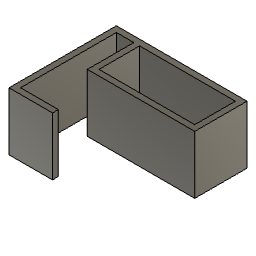
hook for a tee part 2 (Autodesk Fusion 360 design; units mm, degrees)
Autodesk Fusion 360 part; units mm, degrees
sketch "Sketch1" plane through (0, 0, 0) normal (0, 0, 1) x (1, 0, 0)
  line L0 (0, 0) -> (33, 0)
  line L1 (33, 0) -> (33, 14)
  line L2 (33, 14) -> (0, 14)
  line L3 (0, 14) -> (0, 0)
  line L4 (-2, 16) -> (35, 16)
  line L5 (35, 16) -> (35, -2)
  line L6 (35, -2) -> (-2, -2)
  line L7 (-2, -2) -> (-2, 16)
  line L8 (-2, 14) -> (-10, 14)
  line L9 (-10, 14) -> (-10, 16)
  line L10 (-10, 16) -> (-2, 16)
  line L11 (-2, 16) -> (-2, 14)
  line L12 (-10, 14) -> (-8, 14)
  line L13 (-8, 14) -> (-8, -19)
  line L14 (-8, -19) -> (-10, -19)
  line L15 (-10, -19) -> (-10, 14)
  line L16 (-10, -19) -> (5, -19)
  line L17 (5, -19) -> (5, -21)
  line L18 (5, -21) -> (-10, -21)
  line L19 (-10, -21) -> (-10, -19)
  dimension "d1" = 33
  dimension "d2" = 14
  dimension "d3" = 33
  dimension "d4" = 15
  dimension "d5" = 2
  constraint horizontal L0
  constraint vertical L1
  constraint horizontal L2
  constraint vertical L3
  constraint coincident L0.start L3.end
  constraint horizontal L4
  constraint vertical L5
  constraint horizontal L6
  constraint vertical L7
  constraint horizontal L8
  constraint vertical L9
  constraint horizontal L10
  constraint vertical L11
  constraint coincident L7 L8.start
  constraint horizontal L12
  constraint vertical L13
  constraint horizontal L14
  constraint vertical L15
  constraint horizontal L16
  constraint vertical L17
  constraint horizontal L18
  constraint vertical L19
  measures "d1" distance of L0.start L0.end
  measures "d2" distance of L0.start L2.end
  measures "d3" distance of L8.end L14.end
  measures "d4" distance of L14.end L16.end
  measures "d5" distance of L14.end L18.end
extrude "Extrude1" add sketch "Sketch1" along normal blind 20
